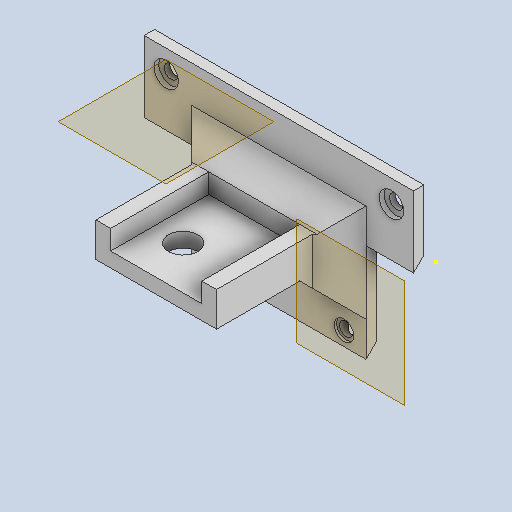
# Autodesk Inventor part: bloco_aquecimento
Saved by Autodesk Inventor 2025.1 (Build 291241000, 241)
## iProperties
Created: 2024-03-21
Part Number: bloco_aquecimento
Material: Genérico
Document SubType Name: Modeling
Designer: joaov
Density: 1 g/cm^3
Appearance: Padrão
Author: joaov
Autodesk Inventor part; units mm, degrees
ref_plane "YZ Plane" through (0, 0, 0) normal (1, 0, 0) x (0, 1, 0)
ref_plane "XZ Plane" through (0, 0, 0) normal (0, 1, 0) x (-1, 0, 0)
ref_plane "XY Plane" through (0, 0, 0) normal (0, 0, 1) x (1, 0, 0)
sketch "Esboço1" plane through (0, 0, 0) normal (0, 0, 1) x (1, 0, 0)
  line L0 (0, 0) -> (0, 15.2)
  line L1 (0, 15.2) -> (-55.362, 15.2)
  line L2 (-55.362, 15.2) -> (-55.362, 0)
  line L3 (-55.362, 0) -> (-45.681, 0)
  line L4 (-45.681, 0) -> (-45.681, -20.1)
  line L5 (-45.681, -20.1) -> (-9.681, -20.1)
  line L6 (-9.681, -20.1) -> (-9.681, 0)
  line L7 (-9.681, 0) -> (0, 0)
  line L8 (-27.681, 15.2) -> (-27.681, 10.2)
  line L9 (-27.681, -20.1) -> (-27.681, -16.9)
  circle A0 centre (-40.981, -16.9) radius 1.4
  circle A1 centre (-50.662, 10.2) radius 1.4
  circle A2 centre (-14.381, -16.9) radius 1.4
  circle A3 centre (-4.7, 10.2) radius 1.4
  dimension "d0" = 15.2
  dimension "d1" = 55.362
  dimension "d2" = 15.2
  dimension "d3" = 9.681
  dimension "d4" = 20.1
  dimension "d5" = 36
  dimension "d6" = 20.1
  dimension "d7" = 5
  dimension "d8" = 3.2
  dimension "d321" = 2.8
  dimension "d322" = 2.8
  dimension "d323" = 2.8
  dimension "d324" = 2.8
  constraints: 20 end point, 4 centre point, 4 perpendicular, 3 vertical, 2 midpoint, 1 horizontal, 1 point on line
  measures "d0" distance of L0.start L0.end
  measures "d1" distance of L0.end L1.end
  measures "d2" distance of L1.end L2.end
  measures "d3" distance of L2.end L3.end
  measures "d4" distance of L3.end L4.end
  measures "d5" distance of L4.end L5.end
  measures "d6" distance of L5.end L6.end
  measures "d7" distance of L8.start L8.end
  measures "d8" distance of L9.start L9.end
  measures "d321" diameter of A0
  measures "d322" diameter of A1
  measures "d323" diameter of A2
  measures "d324" diameter of A3
extrude "Extrusão1" add sketch "Esboço1" along normal blind 4.5
sketch "Esboço21" plane through (0, 0, 4.5) normal (0, 0, 1) x (1, 0, 0)
  line L0 (-55.362, 15.2) -> (-55.362, 0) projected
  line L1 (-55.362, 15.2) -> (-55.262, 15.2)
  line L2 (0, 15.2) -> (-55.362, 15.2) projected
  line L3 (0, 15.2) -> (-55.362, 15.2) projected
  line L4 (0, 15.2) -> (-0.1, 15.2)
  line L5 (-9.681, 0) -> (0, 0) projected
  line L6 (0, 0) -> (-0.1, 0)
  line L7 (-9.681, -20.1) -> (-9.681, 0) projected
  line L8 (-9.681, -20.1) -> (-9.781, -20.1)
  line L9 (-45.681, -20.1) -> (-9.681, -20.1) projected
  line L10 (-45.681, -20.1) -> (-45.581, -20.1)
  line L11 (-45.581, -20.1) -> (-45.681, -20.1)
  line L12 (-45.681, 0) -> (-45.681, -20.1) projected
  line L13 (-55.362, 0) -> (-45.681, 0) projected
  line L14 (-55.362, 0) -> (-55.262, 0)
  line L15 (-55.262, 0.1) -> (-45.581, 0.1)
  line L16 (-45.581, 0.1) -> (-45.581, -20)
  line L17 (-45.581, -20) -> (-9.781, -20)
  line L18 (-9.781, -20) -> (-9.781, 0)
  line L19 (-9.781, 0) -> (-9.781, 0.1)
  line L20 (-9.781, 0.1) -> (-9.681, 0.1)
  line L21 (-9.781, 0.1) -> (-9.681, 0.1)
  line L22 (-9.681, 0.1) -> (-0.1, 0.1)
  line L23 (0, 0) -> (0, 15.2) projected
  line L24 (-0.1, 0.1) -> (-0.1, 15.1)
  line L25 (-0.1, 15.1) -> (-55.262, 15.1)
  line L26 (-55.262, 15.1) -> (-55.262, 0.1)
  line L27 (-55.362, 15.2) -> (-55.362, 0)
  line L28 (-55.362, 0) -> (-45.681, 0)
  line L29 (-45.681, 0) -> (-45.681, -20.1)
  line L30 (-45.681, -20.1) -> (-9.681, -20.1)
  line L31 (-9.681, -20.1) -> (-9.681, 0)
  line L32 (-9.681, 0) -> (0, 0)
  line L33 (0, 0) -> (0, 15.2)
  line L34 (0, 15.2) -> (-55.362, 15.2)
  point P0 (-47.681, 15.2)
  dimension "d203" = 0.1
  dimension "d204" = 0.1
  constraints: 52 end point, 6 perpendicular, 6 point on line, 4 equal length, 2 vertical
  measures "d203" distance of L0.start L1.end
  measures "d204" distance of L1.end L25.end
extrude "rebarba" cut sketch "Esboço21" along normal mid plane 20.5
sketch "Esboço24" plane through (-9.781, -20, 4.5) normal (1, 0, 0) x (0, 0, -1)
  line L0 (2.5, 0.2) -> (4.5, 0.2)
  line L1 (3.4293, 1.2707) -> (4.5, 2.3414)
  line L2 (3.4293, 1.2707) -> (2.3586, 0.2)
  line L3 (4.5, 2.3414) -> (4.5, 0.2)
  line L4 (2.3586, 0.2) -> (4.5, 0.2)
  line L5 (4.5, 2.1414) -> (4.5, 2.3414)
  line L6 (0, 0) -> (0, 20.1) projected
  line L7 (4.5, 0) -> (0, 0)
  line L8 (0, 0) -> (0, 0.2)
  line L9 (0, 0.2) -> (4.5, 0.2)
  line L10 (4.5, 0.2) -> (4.5, 0)
  point P0 (4.5, 20)
  point P1 (4.5, 0.2)
  point P2 (2.3586, 0.2)
  dimension "d270" = 0.2
  constraints: 20 end point, 2 horizontal, 2 parallel, 1 perpendicular, 1 point on line
  measures "d270" distance of L5.start L5.end
extrude "Extrusão18" cut sketch "Esboço24" against normal through all
sketch "Esboço25" plane through (-0.1, 0.1, 4.5) normal (1, 0, 0) x (0, 0, -1)
  line L0 (3.4, 1.2) -> (4.5, 2.3)
  line L1 (3.4, 1.2) -> (2.4, 0.2)
  line L2 (2.4, 0.2) -> (4.5, 0.2)
  line L3 (4.5, 0.2) -> (4.5, 2.3)
  line L4 (4.5, 2.3) -> (3.95, 2.3)
  line L5 (4.899, 0.2) -> (-0.488, 0.2)
  line L6 (-0.488, 0.2) -> (-0.488, 0)
  line L7 (-0.488, 0) -> (4.899, 0)
  line L8 (4.899, 0) -> (4.899, 0.2)
  point P0 (4.5, 0)
  point P1 (2.4, 0.2)
  constraints: 18 end point, 2 horizontal, 2 parallel, 2 perpendicular, 1 point on line
extrude "Extrusão19" cut sketch "Esboço25" against normal blind 9.681
sketch "Esboço26" plane through (-55.262, 0.1, 4.5) normal (-1, 0, 0) x (0, 0, 1)
  line L0 (-4.5, 2.3) -> (-2.4, 0.2)
  line L1 (-4.5, 0.2) -> (-2.4, 0.2)
  line L2 (-4.5, 0.2) -> (-2.4, 0.2)
  line L3 (-4.5, 2.3) -> (-4.5, 0.2)
  line L4 (-4.5, 0) -> (-4.5, -17.7586) projected
  line L5 (-4.5, 0) -> (-4.5, 15) projected
  line L6 (-4.5, 2.3) -> (-4.3, 2.3)
  line L7 (-4.7094, 0.2) -> (0.2738, 0.2)
  line L8 (0.2738, 0.2) -> (0.2738, 0)
  line L9 (0.2738, 0) -> (-4.7094, 0)
  line L10 (-4.7094, 0) -> (-4.7094, 0.2)
  point P0 (-2.4, 0.2)
  constraints: 18 end point, 3 horizontal, 2 collinear, 2 parallel, 1 perpendicular, 1 point on line
extrude "Extrusão20" cut sketch "Esboço26" against normal blind 9.681
ref_plane "Plano de trabalho3" through (0, 0, 17.5) normal (0, 0, 1) x (1, 0, 0)
sketch "Esboço27" plane through (0, 0, 17.5) normal (0, 0, 1) x (1, 0, 0)
  line L0 (-55.262, 15.1) -> (-55.262, 14.8)
  line L1 (-55.262, 14.8) -> (-0.1, 14.8)
  line L2 (-0.1, 14.8) -> (-55.262, 14.8)
  line L3 (-55.262, 14.8) -> (-55.262, 15.7059)
  line L4 (-55.262, 15.7059) -> (-0.1, 15.7059)
  line L5 (-0.1, 15.7059) -> (-0.1, 14.8)
  point P0 (0, 0)
  dimension "d274" = 90
  constraints: 12 end point, 2 parallel, 1 horizontal, 1 perpendicular
  measures "d274" angle of L1 L0
extrude "Extrusão21" cut sketch "Esboço27" against normal through all
ref_plane "Plano de trabalho2" through (-37.681, 14.8, 17.5) normal (0, 1, 0) x (1, 0, 0)
sketch "Esboço28" plane through (-37.681, 14.8, 17.5) normal (0, 1, 0) x (1, 0, 0)
  line L0 (-17.581, 17.5) -> (-17.481, 17.5)
  line L1 (-17.481, 17.5) -> (-17.481, 12.5734)
  line L2 (-17.481, 17.5) -> (-17.7304, 17.5)
  line L3 (-17.7304, 17.5) -> (-17.7304, 12.8429)
  line L4 (-17.7304, 12.8429) -> (-17.481, 12.8429)
  line L5 (-17.481, 12.8429) -> (-17.481, 17.5)
  line L6 (10, 17.5) -> (10, 11.5745)
  line L7 (37.581, 17.5) -> (37.481, 17.5)
  line L8 (37.481, 17.5) -> (37.481, 12.5734)
  line L9 (37.481, 17.5) -> (37.7304, 17.5)
  line L10 (37.7304, 17.5) -> (37.7304, 12.8429)
  line L11 (37.7304, 12.8429) -> (37.481, 12.8429)
  line L12 (37.481, 12.8429) -> (37.481, 17.5)
  point P0 (37.681, 17.5)
  point P1 (-17.481, 12.8429)
  constraints: 26 end point, 5 symmetric about line, 2 parallel, 2 perpendicular, 1 horizontal, 1 vertical
extrude "Extrusão22" cut sketch "Esboço28" against normal through all
sketch "Esboço29" plane through (-9.781, -19.8, 2.1414) normal (0, -1, 0) x (1, 0, 0)
  line L0 (0, 0) -> (0, -2.1414) projected
  line L1 (0, 0) -> (-0.1, 0)
  line L2 (0, 0) -> (-35.8, 0) projected
  line L3 (-0.1, 0) -> (-0.1, -2.4621)
  line L4 (-0.1, 0) -> (-0.1, 2.728)
  line L5 (-0.1, 2.728) -> (0.1398, 2.728)
  line L6 (0.1398, 2.728) -> (0.1398, -2.4621)
  line L7 (0.1398, -2.4621) -> (-0.1, -2.4621)
  line L8 (-0.1, -2.4621) -> (-0.1, 2.728)
  line L9 (-17.9, 0) -> (-17.9, -4.1402)
  line L10 (-35.8, 0) -> (-35.8, -2.1414)
  line L11 (-35.8, 0) -> (-35.7, 0)
  line L12 (-35.7, 0) -> (-35.7, -2.4621)
  line L13 (-35.7, 0) -> (-35.7, 2.728)
  line L14 (-35.7, 2.728) -> (-35.9398, 2.728)
  line L15 (-35.9398, 2.728) -> (-35.9398, -2.4621)
  line L16 (-35.9398, -2.4621) -> (-35.7, -2.4621)
  line L17 (-35.7, -2.4621) -> (-35.7, 2.728)
  point P0 (9.781, -2.1414)
  point P1 (-0.1, -2.4621)
  dimension "d280" = 0.1
  constraints: 32 end point, 7 symmetric about line, 3 vertical, 2 parallel, 1 horizontal, 1 midpoint, 1 perpendicular, 1 point on line
  measures "d280" distance of L0.start L1.end
extrude "Extrusão23" cut sketch "Esboço29" against normal blind 20.1
sketch "Esboço30" plane through (-45.581, 0.3, 0) normal (-1, 0, 0) x (0, 0, 1)
  line L0 (0, 0) -> (0, 2.1) projected
  line L1 (0, 2.1) -> (0, 0)
  line L2 (0, 2.1) -> (2.1, 0) projected
  line L3 (0, 0) -> (2.1, 0)
  line L4 (2.1, 0) -> (0, 2.1)
  constraints: 6 end point, 2 collinear, 1 horizontal
extrude "Extrusão24" cut sketch "Esboço30" against normal blind 0.1
sketch "Esboço31" plane through (-9.781, 0.3, 0) normal (1, 0, 0) x (0, 0, -1)
  line L0 (-2.1, 0) -> (0, 2.1) projected
  line L1 (0, 2.1) -> (-2.1, 0)
  line L2 (0, 0) -> (-4.5, 0) projected
  line L3 (-2.1, 0) -> (0, 0)
  line L4 (0, 0) -> (0, 2.1)
  point P0 (0, -0.3)
  constraints: 6 end point, 2 collinear, 1 perpendicular
extrude "Extrusão25" cut sketch "Esboço31" against normal blind 0.1
sketch "Esboço35" plane through (0, 0, 4.5) normal (0, 0, 1) x (1, 0, 0)
  line L0 (-9.881, 0.3) -> (-0.2, 0.3) projected
  line L1 (-45.481, 0.3) -> (-45.481, -19.8) projected
  line L2 (-9.881, 0.3) -> (-45.481, 0.3)
  line L3 (-27.681, 0.3) -> (-27.681, 2.3)
  line L4 (-27.681, 0.3) -> (-27.681, -1.7)
  line L5 (-27.681, -1.7) -> (-36.981, -1.7)
  line L6 (-27.681, -1.7) -> (-18.381, -1.7)
  line L7 (-36.981, -1.7) -> (-18.381, -1.7)
  line L8 (-18.381, -1.7) -> (-18.381, 2.3)
  line L9 (-18.381, 2.3) -> (-36.981, 2.3)
  line L10 (-36.981, 2.3) -> (-36.981, -1.7)
  point P0 (0, 0)
  constraints: 18 end point, 3 horizontal, 3 parallel, 2 vertical, 1 midpoint, 1 perpendicular
extrude "Extrusão26" add sketch "Esboço35" along normal blind 5
sketch "Esboço37" plane through (0, 0, 4.5) normal (0, 0, 1) x (1, 0, 0)
  line L0 (-36.981, 2.3) -> (-18.381, 2.3) projected
  line L1 (-36.981, 2.3) -> (-39.981, 2.3)
  line L2 (-39.981, 2.3) -> (-39.981, -2.7)
  line L3 (-39.981, -2.7) -> (-39.981, -4.7)
  line L4 (-39.981, -4.7) -> (-18.381, -4.7)
  line L5 (-18.381, -4.7) -> (-15.381, -4.7)
  line L6 (-15.381, -4.7) -> (-15.381, 2.3)
  line L7 (-18.381, 2.3) -> (-18.381, -1.7) projected
  line L8 (-15.381, 2.3) -> (-18.381, 2.3)
  line L9 (-18.381, 2.3) -> (-18.381, -1.7)
  line L10 (-36.981, -1.7) -> (-36.981, 2.3) projected
  line L11 (-18.381, -1.7) -> (-36.981, -1.7)
  line L12 (-36.981, -1.7) -> (-36.981, 2.3)
  point P0 (0, 0)
  dimension "d297" = 3
  dimension "d298" = 5
  dimension "d299" = 2
  dimension "d300" = 3
  constraints: 20 end point, 7 perpendicular, 3 point on line, 1 horizontal
  measures "d297" distance of L0.start L1.end
  measures "d298" distance of L1.end L2.end
  measures "d299" distance of L2.end L3.end
  measures "d300" distance of L4.end L5.end
extrude "Extrusão27" add sketch "Esboço37" along normal blind 25 contours L10 L11 L7 L8 L6 L5 L4 L3 L2 L1
sketch "Esboço38" plane through (-36.981, -1.7, 9.5) normal (0, 1, 0) x (1, 0, 0)
  line L0 (0, -20) -> (6, -20)
  circle A0 centre (6, -11.2) radius 3
  line L1 (0, 0) -> (0, -20) projected
  point P0 (36.981, 9.5)
  dimension "d306" = 6
  dimension "d307" = 8.8
  constraints: 2 end point, 1 centre point
  measures "d306" distance from line of L1 A0.centre
  measures "d307" distance of L0.end A0.centre
extrude "Extrusão28" cut sketch "Esboço38" against normal through all
chamfer "Chanfro5" distance 5 angle 45 1 edges at (-27.681, 2.3, 4.5)
chamfer "Chanfro6" distance 5.5 angle 45 4 edges at (-39.981, 4.8, 4.5) (-39.981, -1.2, 4.5) (-15.381, 4.8, 4.5) (-15.381, -1.2, 4.5)
chamfer "Chanfro7" distance 8 angle 45 1 edges at (-27.681, -4.7, 4.5)
sketch "Esboço39" plane through (-0.2, 0.3, 4.5) normal (1, 0, 0) x (0, 0, -1)
  line L0 (4.5, 14.5) -> (4.5, 2.1) projected
  line L1 (4.4982, 14.5) -> (-0.0018, 14.5)
  line L2 (0, -20.1) -> (2.1414, -17.9586)
  line L3 (2.1414, -17.9586) -> (2.1414, -20.1)
  line L4 (2.1414, -20.1) -> (0, -20.1)
  line L5 (2.1414, -17.9586) -> (2.1414, 18.9845)
  line L6 (2.1414, 18.9845) -> (5.2102, 18.9845)
  line L7 (5.2102, 18.9845) -> (5.2102, -20.1)
  line L8 (5.2102, -20.1) -> (2.1414, -20.1)
  line L9 (2.1414, -20.1) -> (2.1414, 18.9845)
  line L10 (0, -20.1) -> (0, -13) projected
  line L11 (0, -20.1) -> (0, -20.0982)
  point P0 (4.5, -0.3)
  point P1 (4.5, -17.9586)
  dimension "d330" = 4.5018
  constraints: 20 end point, 3 perpendicular, 2 parallel, 1 horizontal, 1 point on line
  measures "d330" distance of L0.start L1.end
extrude "Extrusão29" cut sketch "Esboço39" against normal through all
sketch "Esboço42" plane through (0, 0, 4.5) normal (0, 0, 1) x (1, 0, 0)
  circle A0 centre (-4.7, 10.2) radius 1.4 projected
  circle A1 centre (-4.7, 10.2) radius 1.4
  circle A2 centre (-4.7, 10.2) radius 2.5
  circle A3 centre (-50.662, 10.2) radius 1.4 projected
  circle A4 centre (-50.662, 10.2) radius 1.4
  circle A5 centre (-50.662, 10.2) radius 2.5
  point P0 (0, 0)
  dimension "d337" = 5
  dimension "d338" = 5
  constraints: 4 centre point, 4 coincident
  measures "d337" diameter of A2
  measures "d338" diameter of A5
extrude "Extrusão32" cut sketch "Esboço42" against normal blind 1
sketch "Esboço43" plane through (0, 0, 4.5) normal (0, 0, 1) x (1, 0, 0)
  circle A0 centre (-40.981, -16.9) radius 1.4 projected
  circle A1 centre (-40.981, -16.9) radius 1.4
  circle A2 centre (-40.981, -16.9) radius 2
  circle A3 centre (-14.381, -16.9) radius 1.4 projected
  circle A4 centre (-14.381, -16.9) radius 1.4
  circle A5 centre (-14.381, -16.9) radius 2
  point P0 (0, 0)
  dimension "d341" = 4
  dimension "d342" = 4
  constraints: 4 centre point, 4 coincident
  measures "d341" diameter of A2
  measures "d342" diameter of A5
extrude "Extrusão33" cut sketch "Esboço43" against normal blind 0.5
sketch "Esboço45" plane through (-0.2, 0.3, 4.5) normal (1, 0, 0) x (0, 0, -1)
  point P0 (4.5, -0.3)
sketch "Esboço46" plane through (-0.2, 0.3, 4.5) normal (1, 0, 0) x (0, 0, -1)
  line L0 (0, -13) -> (0, -20.1) projected
  line L1 (2.1414, 2.1414) -> (0, 0)
  line L2 (0, 0) -> (2.1414, 0)
  line L3 (2.1414, 0) -> (2.1414, 2.1414)
  line L4 (0, 0) -> (2.1414, 0) projected
  line L5 (0, 0) -> (2.1414, 0)
  point P0 (4.5, -0.3)
  point P1 (2.1414, -17.9586)
  constraints: 8 end point, 2 perpendicular, 1 collinear
extrude "Extrusão34" cut sketch "Esboço46" against normal blind 9.681
sketch "Esboço47" plane through (-55.162, 0.3, 4.5) normal (-1, 0, 0) x (0, 0, 1)
  line L0 (0, -20.1) -> (-2.1414, -17.9586) projected
  line L1 (-2.1414, -17.9586) -> (0, -20.1)
  line L2 (0, -20.1) -> (-2.1414, -20.1)
  line L3 (-2.1414, -20.1) -> (-2.1414, -17.9586)
  line L4 (0, 0) -> (-2.1414, 2.1414) projected
  line L5 (0, -13) -> (0, 0) projected
  line L6 (-2.1414, 2.1414) -> (0, 0)
  line L7 (0, 0) -> (-2.1414, 0)
  line L8 (-2.1414, 0) -> (-2.1414, 2.1414)
  constraints: 12 end point, 3 perpendicular, 1 collinear, 1 horizontal
extrude "Extrusão35" cut sketch "Esboço47" against normal blind 9.681 contours L7 L8 L4
